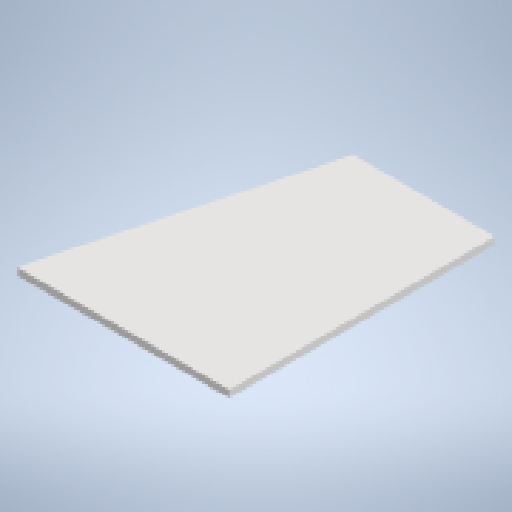
# Autodesk Inventor part: держатель полки 1
Saved by Autodesk Inventor 2025 (Build 290162010, 162A)
## iProperties
Created: 2024-06-15
Part Number: держатель полки 1
Material: Generic
Document SubType Name: Sheet Metal
Designer: admin
Density: 1 g/cm^3
Sheet Metal Rule: Default
Appearance: Default
Author: admin
Autodesk Inventor part; units mm, degrees
ref_plane "YZ Plane" through (0, 0, 0) normal (1, 0, 0) x (0, 1, 0)
ref_plane "XZ Plane" through (0, 0, 0) normal (0, 1, 0) x (-1, 0, 0)
ref_plane "XY Plane" through (0, 0, 0) normal (0, 0, 1) x (1, 0, 0)
sketch "Sketch1" plane through (0, 0, 0) normal (0, 0, 1) x (1, 0, 0)
  line L0 (-160, 0) -> (0, 0)
  line L1 (-160, -300) -> (-160, 0) construction
  line L2 (-160, 0) -> (-240.3848, -300)
  line L3 (-240.3848, -300) -> (-160, -300)
  line L4 (0, 0) -> (-80.3848, -300) construction
  line L5 (0, 0) -> (160, 0)
  line L6 (0, 0) -> (0, -300)
  line L7 (0, -300) -> (-160, -300)
  dimension "d2" = 15
  dimension "d29" = 160
  dimension "d40" = 300
  dimension "d41" = 15
  measures "d2" angle of L1 L2
  measures "d29" distance of L4.end L2.end
  measures "d40" distance between parallel lines of L7 L0
  measures "d41" angle of L6 L4
extrude "Plate1" add sketch "Sketch1" along normal blind 8
fillet "Corner Round1" radius 2 3 edges at (-240.3848, -300, 4) (0, 0, 4) (-160, 0, 4)
equation "\"d3\" = Thickness"
equation "\"BendRadius\" = Thickness"
equation "\"BendReliefWidth\" = Thickness"
equation "\"BendReliefDepth\" = 0.5 * Thickness"
equation "\"CornerReliefSize\" = 4 * Thickness"
equation "\"MinimumRemnant\" = 2 * Thickness"
equation "\"TransitionRadius\" = BendRadius"
equation "\"JacobiRadiusSize\" = BendRadius"
equation "\"GapSize\" = Thickness"
equation "\"Thickness\" = 8"
body "Solid1"
